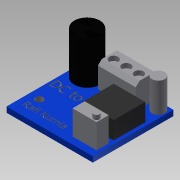
# Autodesk Inventor part: DC to DC
Saved by Autodesk Inventor 2015 SP1 (Build 190203100, 203)
## iProperties
Created: 2015-01-28
Part Number: DC to DC
Material: Generic
Document SubType Name: Modeling
Designer: Rafi Kurnia Putra
Density: 1 g/cm^3
Appearance: Default
Mass: 6.54094 g
Surface Area: 45.9552 cm^2
Volume: 6.54094 cm^3
Author: Rafi Kurnia Putra
Autodesk Inventor part; units mm, degrees
ref_plane "YZ Plane" through (0, 0, 0) normal (1, 0, 0) x (0, 1, 0)
ref_plane "XZ Plane" through (0, 0, 0) normal (0, 1, 0) x (-1, 0, 0)
ref_plane "XY Plane" through (0, 0, 0) normal (0, 0, 1) x (1, 0, 0)
sketch "Sketch1" plane through (0, 0, 0) normal (0, 1, 0) x (-1, 0, 0)
  line L0 (17.14, 16) -> (-17.14, 16)
  line L1 (-17.14, 16) -> (-17.14, -16)
  line L2 (-17.14, -16) -> (17.14, -16)
  line L3 (17.14, -16) -> (17.14, 16)
  line L4 (17.14, 16) -> (-17.14, -16) construction
  line L5 (-17.14, 16) -> (17.14, -16) construction
  circle A0 centre (13.09, 7.05) radius 1.5
  circle A1 centre (11.14, -10) radius 5.065
  circle A2 centre (2.4487, -11.859) radius 1.75
  circle A3 centre (-2.5513, -11.859) radius 1.75
  circle A4 centre (-7.5513, -11.859) radius 1.75
  circle A5 centre (-14.14, -13) radius 2.5
  line L6 (-3.3092, -6.109) -> (-15.8092, -6.109)
  line L7 (-15.8092, -6.109) -> (-15.8092, 6.391)
  line L8 (-15.8092, 6.391) -> (-3.3092, 6.391)
  line L9 (-3.3092, 6.391) -> (-3.3092, -6.109)
  line L10 (-3.3092, -6.109) -> (-15.8092, 6.391) construction
  line L11 (-15.8092, -6.109) -> (-3.3092, 6.391) construction
  line L12 (4.9487, -15.609) -> (-10.0513, -15.609)
  line L13 (-10.0513, -15.609) -> (-10.0513, -8.109)
  line L14 (-10.0513, -8.109) -> (4.9487, -8.109)
  line L15 (4.9487, -8.109) -> (4.9487, -15.609)
  line L16 (4.9487, -15.609) -> (-10.0513, -8.109) construction
  line L17 (-10.0513, -15.609) -> (4.9487, -8.109) construction
  line L18 (-6.279, 8.3837) -> (-15.809, 8.3837)
  line L19 (-15.809, 8.3837) -> (-15.809, 13.2037)
  line L20 (-15.809, 13.2037) -> (-6.279, 13.2037)
  line L21 (-6.279, 13.2037) -> (-6.279, 8.3837)
  line L22 (-6.279, 8.3837) -> (-15.809, 13.2037) construction
  line L23 (-15.809, 8.3837) -> (-6.279, 13.2037) construction
  circle A6 centre (-14.309, 11.7037) radius 1.155
  point P0 (0, 0)
  point P1 (-9.5592, 0.141)
  point P2 (-2.5513, -11.859)
  point P3 (-11.044, 10.7937)
  point P4 (-9.5592, 0.141)
  dimension "d0" = 34.28
  dimension "d1" = 32
  dimension "d2" = 3
  dimension "d3" = 4.05
  dimension "d4" = 8.95
  dimension "d5" = 10.13
  dimension "d6" = 6
  dimension "d7" = 6
  dimension "d8" = 3.5
  dimension "d9" = 3.5
  dimension "d10" = 3.5
  dimension "d11" = 5
  dimension "d12" = 5
  dimension "d13" = 5
  dimension "d14" = 3
  dimension "d15" = 3
  dimension "d16" = 12.5
  dimension "d17" = 12.5
  dimension "d18" = 15
  dimension "d19" = 7.5
  dimension "d20" = 2
  dimension "d21" = 9.53
  dimension "d22" = 4.82
  dimension "d23" = 1.3308
  dimension "d24" = 1.331
  dimension "d42" = 2.31
  dimension "d43" = 1.5
  dimension "d44" = 1.5
  constraints: 48 end point, 9 midpoint, 8 parallel, 7 centre point, 4 horizontal, 4 perpendicular, 1 other
  measures "d0" distance of L2.end L1.end
  measures "d1" distance of L1.end L0.end
  measures "d2" diameter of A0
  measures "d3" distance from line of A0.centre L3
  measures "d4" distance from line of L0 A0.centre
  measures "d5" diameter of A1
  measures "d6" distance from line of A1.centre L3
  measures "d7" distance from line of L2 A1.centre
  measures "d8" diameter of A2
  measures "d9" diameter of A3
  measures "d10" diameter of A4
  measures "d11" distance of A3.centre A2.centre
  measures "d12" distance of A4.centre A3.centre
  measures "d13" diameter of A5
  measures "d14" distance from line of A5.centre L2
  measures "d15" distance from line of L1 A5.centre
  measures "d16" distance of L7.end L8.end
  measures "d17" distance of L6.end L7.end
  measures "d18" distance of L13.end L14.end
  measures "d19" distance of L12.end L13.end
  measures "d20" distance between parallel lines of L6 L14
  measures "d21" distance of L19.end L20.end
  measures "d22" distance of L18.end L19.end
  measures "d23" distance between parallel lines of L1 L7
  measures "d24" distance between parallel lines of L1 L19
  measures "d42" diameter of A6
  measures "d43" distance from line of A6.centre L20
  measures "d44" distance from line of L19 A6.centre
extrude "Extrusion1" add sketch "Sketch1" along normal blind 2.15 contours L3 L2 L1 L0 | A1 | A2 | A3 | A4 | A5 | L6 L7 L8 L9 | L12 L13 L14 L15 | L18 L19 L20 L21 | A6
extrude "Extrusion2" add sketch "Sketch1" along normal blind 19.17 contours A1
extrude "Extrusion3" add sketch "Sketch1" along normal blind 11.77 contours L12 L13 L14 L15
chamfer "Chamfer1" distance 1.5 angle 45 1 edges at (2.5513, 11.77, -8.109)
extrude "Extrusion4" add sketch "Sketch1" along normal blind 10 contours A2 | A3 | A4
extrude "Extrusion5" add sketch "Sketch1" along normal blind 13.91 contours A5
extrude "Extrusion6" add sketch "Sketch1" along normal blind 9.14 contours L6 L7 L8 L9
extrude "Extrusion7" add sketch "Sketch1" along normal blind 11.85 contours L18 L19 L20 L21 | A6
extrude "Extrusion8" add sketch "Sketch1" along normal blind 13.61 contours A6
extrude "Extrusion9" add sketch "Sketch1" against normal blind 2.4 contours A2 | A3 | A4
sketch "Sketch2" plane through (0, 2.15, 0) normal (0, 1, 0) x (1, 0, 0)
  line L0 (-16.4252, 3.2471) -> (3.1141, 3.2471) construction
  line L1 (3.1141, 3.2471) -> (3.1141, -0.3891) construction
  line L2 (3.1141, -0.3891) -> (-16.4252, -0.3891) construction
  line L3 (-16.4252, -0.3891) -> (-16.4252, 3.2471) construction
  line L4 (-14.8497, -9.856) -> (21.0749, -9.856) construction
  line L5 (21.0749, -9.856) -> (21.0749, -13.6084) construction
  line L6 (21.0749, -13.6084) -> (-14.8497, -13.6084) construction
  line L7 (-14.8497, -13.6084) -> (-14.8497, -9.856) construction
  line L8 (-12.6267, -12.5257) -> (-13.0651, -12.5257)
  line L9 (-13.0651, -12.5257) -> (-13.8679, -11.515)
  line L10 (-13.8679, -11.515) -> (-14.2549, -11.515)
  line L11 (-14.2549, -11.515) -> (-14.2549, -12.5257)
  line L12 (-14.2549, -12.5257) -> (-14.5924, -12.5257)
  line L13 (-14.5924, -12.5257) -> (-14.5924, -9.9857)
  line L14 (-14.5924, -9.9857) -> (-13.9379, -9.9857)
  spline S0 degree 2 poles (-13.9379, -9.9857) (-13.7197, -9.9857) (-13.4253, -10.033) (-13.2916, -10.1195) knots 0 0 0 1 2 2 2
  spline S1 degree 2 poles (-13.2916, -10.1195) (-13.1578, -10.2059) (-13.0034, -10.4756) (-13.0034, -10.6752) knots 0 0 0 1 2 2 2
  spline S2 degree 2 poles (-13.0034, -10.6752) (-13.0034, -10.9531) (-13.2874, -11.3298) (-13.5303, -11.4204) knots 0 0 0 1 2 2 2
  line L15 (-13.5303, -11.4204) -> (-12.6267, -12.5257)
  spline S3 degree 2 poles (-13.3554, -10.702) (-13.3554, -10.5908) (-13.4336, -10.42) (-13.5159, -10.3644) knots 0 0 0 1 2 2 2
  spline S4 degree 2 poles (-13.5159, -10.3644) (-13.588, -10.3171) (-13.7794, -10.278) (-13.9193, -10.278) knots 0 0 0 1 2 2 2
  line L16 (-13.9193, -10.278) -> (-14.2549, -10.278)
  line L17 (-14.2549, -10.278) -> (-14.2549, -11.233)
  line L18 (-14.2549, -11.233) -> (-13.9585, -11.233)
  spline S5 degree 2 poles (-13.9585, -11.233) (-13.8123, -11.233) (-13.5797, -11.1816) (-13.4994, -11.1013) knots 0 0 0 1 2 2 2
  spline S6 degree 2 poles (-13.4994, -11.1013) (-13.4253, -11.0313) (-13.3554, -10.8337) (-13.3554, -10.702) knots 0 0 0 1 2 2 2
  spline S7 degree 2 poles (-11.3876, -12.324) (-11.4267, -12.3528) (-11.5584, -12.4557) (-11.6202, -12.4866) knots 0 0 0 1 2 2 2
  spline S8 degree 2 poles (-11.6202, -12.4866) (-11.7046, -12.5319) (-11.8631, -12.5792) (-12.0071, -12.5792) knots 0 0 0 1 2 2 2
  spline S9 degree 2 poles (-12.0071, -12.5792) (-12.1245, -12.5792) (-12.3365, -12.4907) (-12.4168, -12.4104) knots 0 0 0 1 2 2 2
  spline S10 degree 2 poles (-12.4168, -12.4104) (-12.4929, -12.3322) (-12.5855, -12.1017) (-12.5855, -11.974) knots 0 0 0 1 2 2 2
  spline S11 degree 2 poles (-12.5855, -11.974) (-12.5855, -11.7764) (-12.4188, -11.4965) (-12.2377, -11.4162) knots 0 0 0 1 2 2 2
  spline S12 degree 2 poles (-12.2377, -11.4162) (-12.0771, -11.3421) (-11.6408, -11.2866) (-11.3876, -11.2722) knots 0 0 0 1 2 2 2
  line L19 (-11.3876, -11.2722) -> (-11.3876, -11.2104)
  spline S13 degree 2 poles (-11.3876, -11.2104) (-11.3876, -11.0993) (-11.4555, -10.9613) (-11.5173, -10.9222) knots 0 0 0 1 2 2 2
  spline S14 degree 2 poles (-11.5173, -10.9222) (-11.579, -10.8831) (-11.756, -10.8584) (-11.8507, -10.8584) knots 0 0 0 1 2 2 2
  spline S15 degree 2 poles (-11.8507, -10.8584) (-11.9619, -10.8584) (-12.2624, -10.9243) (-12.4126, -10.9881) knots 0 0 0 1 2 2 2
  line L20 (-12.4126, -10.9881) -> (-12.4312, -10.9881)
  line L21 (-12.4312, -10.9881) -> (-12.4312, -10.6608)
  spline S16 degree 2 poles (-12.4312, -10.6608) (-12.3427, -10.6361) (-12.0113, -10.5744) (-11.8486, -10.5744) knots 0 0 0 1 2 2 2
  spline S17 degree 2 poles (-11.8486, -10.5744) (-11.651, -10.5744) (-11.3814, -10.6361) (-11.2744, -10.7164) knots 0 0 0 1 2 2 2
  spline S18 degree 2 poles (-11.2744, -10.7164) (-11.1694, -10.7946) (-11.0665, -11.0437) (-11.0665, -11.2228) knots 0 0 0 1 2 2 2
  line L22 (-11.0665, -11.2228) -> (-11.0665, -12.5257)
  line L23 (-11.0665, -12.5257) -> (-11.3876, -12.5257)
  line L24 (-11.3876, -12.5257) -> (-11.3876, -12.324)
  line L25 (-11.3876, -12.0564) -> (-11.3876, -11.5274)
  spline S19 degree 2 poles (-11.3876, -11.5274) (-11.5028, -11.5377) (-11.8507, -11.5727) (-11.9598, -11.6056) knots 0 0 0 1 2 2 2
  spline S20 degree 2 poles (-11.9598, -11.6056) (-12.0874, -11.6447) (-12.2541, -11.8073) (-12.2541, -11.9514) knots 0 0 0 1 2 2 2
  spline S21 degree 2 poles (-12.2541, -11.9514) (-12.2541, -12.1161) (-12.0689, -12.2828) (-11.8919, -12.2828) knots 0 0 0 1 2 2 2
  spline S22 degree 2 poles (-11.8919, -12.2828) (-11.7416, -12.2828) (-11.4946, -12.1531) (-11.3876, -12.0564) knots 0 0 0 1 2 2 2
  line L26 (-9.6133, -10.1812) -> (-9.6298, -10.1812)
  spline S23 degree 2 poles (-9.6298, -10.1812) (-9.673, -10.1648) (-9.8335, -10.1359) (-9.8973, -10.1359) knots 0 0 0 1 2 2 2
  spline S24 degree 2 poles (-9.8973, -10.1359) (-10.0991, -10.1359) (-10.272, -10.3171) (-10.272, -10.5558) knots 0 0 0 1 2 2 2
  line L27 (-10.272, -10.5558) -> (-10.272, -10.6197)
  line L28 (-10.272, -10.6197) -> (-9.7409, -10.6197)
  line L29 (-9.7409, -10.6197) -> (-9.7409, -10.8852)
  line L30 (-9.7409, -10.8852) -> (-10.2617, -10.8852)
  line L31 (-10.2617, -10.8852) -> (-10.2617, -12.5257)
  line L32 (-10.2617, -12.5257) -> (-10.5828, -12.5257)
  line L33 (-10.5828, -12.5257) -> (-10.5828, -10.8852)
  line L34 (-10.5828, -10.8852) -> (-10.7989, -10.8852)
  line L35 (-10.7989, -10.8852) -> (-10.7989, -10.6197)
  line L36 (-10.7989, -10.6197) -> (-10.5828, -10.6197)
  line L37 (-10.5828, -10.6197) -> (-10.5828, -10.5558)
  spline S25 degree 2 poles (-10.5828, -10.5558) (-10.5828, -10.2142) (-10.2514, -9.856) (-9.9426, -9.856) knots 0 0 0 1 2 2 2
  spline S26 degree 2 poles (-9.9426, -9.856) (-9.8541, -9.856) (-9.6833, -9.8745) (-9.6133, -9.8869) knots 0 0 0 1 2 2 2
  line L38 (-9.6133, -9.8869) -> (-9.6133, -10.1812)
  line L39 (-9.1769, -12.5257) -> (-9.498, -12.5257)
  line L40 (-9.498, -12.5257) -> (-9.498, -10.6197)
  line L41 (-9.498, -10.6197) -> (-9.1769, -10.6197)
  line L42 (-9.1769, -10.6197) -> (-9.1769, -12.5257)
  line L43 (-9.1543, -10.3027) -> (-9.5186, -10.3027)
  line L44 (-9.5186, -10.3027) -> (-9.5186, -9.9692)
  line L45 (-9.5186, -9.9692) -> (-9.1543, -9.9692)
  line L46 (-9.1543, -9.9692) -> (-9.1543, -10.3027)
  line L47 (-5.7374, -12.5257) -> (-6.1758, -12.5257)
  line L48 (-6.1758, -12.5257) -> (-7.1042, -11.3442)
  line L49 (-7.1042, -11.3442) -> (-7.2524, -11.5109)
  line L50 (-7.2524, -11.5109) -> (-7.2524, -12.5257)
  line L51 (-7.2524, -12.5257) -> (-7.5899, -12.5257)
  line L52 (-7.5899, -12.5257) -> (-7.5899, -9.9857)
  line L53 (-7.5899, -9.9857) -> (-7.2524, -9.9857)
  line L54 (-7.2524, -9.9857) -> (-7.2524, -11.1528)
  line L55 (-7.2524, -11.1528) -> (-6.2108, -9.9857)
  line L56 (-6.2108, -9.9857) -> (-5.7992, -9.9857)
  line L57 (-5.7992, -9.9857) -> (-6.851, -11.1198)
  line L58 (-6.851, -11.1198) -> (-5.7374, -12.5257)
  line L59 (-4.0784, -12.5257) -> (-4.3995, -12.5257)
  line L60 (-4.3995, -12.5257) -> (-4.3995, -12.3157)
  spline S27 degree 2 poles (-4.3995, -12.3157) (-4.5477, -12.4454) (-4.8132, -12.5792) (-4.9779, -12.5792) knots 0 0 0 1 2 2 2
  spline S28 degree 2 poles (-4.9779, -12.5792) (-5.1014, -12.5792) (-5.3216, -12.4969) (-5.4019, -12.4084) knots 0 0 0 1 2 2 2
  spline S29 degree 2 poles (-5.4019, -12.4084) (-5.4842, -12.3199) (-5.5748, -12.0502) (-5.5748, -11.8567) knots 0 0 0 1 2 2 2
  line L61 (-5.5748, -11.8567) -> (-5.5748, -10.6197)
  line L62 (-5.5748, -10.6197) -> (-5.2537, -10.6197)
  line L63 (-5.2537, -10.6197) -> (-5.2537, -11.7065)
  spline S30 degree 2 poles (-5.2537, -11.7065) (-5.2537, -11.8588) (-5.2311, -12.0584) (-5.192, -12.1325) knots 0 0 0 1 2 2 2
  spline S31 degree 2 poles (-5.192, -12.1325) (-5.1528, -12.2066) (-5.0191, -12.2746) (-4.8935, -12.2746) knots 0 0 0 1 2 2 2
  spline S32 degree 2 poles (-4.8935, -12.2746) (-4.7762, -12.2746) (-4.5106, -12.1408) (-4.3995, -12.044) knots 0 0 0 1 2 2 2
  line L64 (-4.3995, -12.044) -> (-4.3995, -10.6197)
  line L65 (-4.3995, -10.6197) -> (-4.0784, -10.6197)
  line L66 (-4.0784, -10.6197) -> (-4.0784, -12.5257)
  line L67 (-2.6026, -10.9634) -> (-2.619, -10.9634)
  spline S33 degree 2 poles (-2.619, -10.9634) (-2.6561, -10.9531) (-2.7363, -10.949) (-2.7919, -10.949) knots 0 0 0 1 2 2 2
  spline S34 degree 2 poles (-2.7919, -10.949) (-2.9216, -10.949) (-3.1768, -11.0622) (-3.2921, -11.1734) knots 0 0 0 1 2 2 2
  line L68 (-3.2921, -11.1734) -> (-3.2921, -12.5257)
  line L69 (-3.2921, -12.5257) -> (-3.6132, -12.5257)
  line L70 (-3.6132, -12.5257) -> (-3.6132, -10.6197)
  line L71 (-3.6132, -10.6197) -> (-3.2921, -10.6197)
  line L72 (-3.2921, -10.6197) -> (-3.2921, -10.9037)
  spline S35 degree 2 poles (-3.2921, -10.9037) (-3.1171, -10.7473) (-2.8557, -10.6197) (-2.7322, -10.6197) knots 0 0 0 1 2 2 2
  spline S36 degree 2 poles (-2.7322, -10.6197) (-2.6828, -10.6197) (-2.6334, -10.6238) (-2.6026, -10.6299) knots 0 0 0 1 2 2 2
  line L73 (-2.6026, -10.6299) -> (-2.6026, -10.9634)
  line L74 (-0.8571, -12.5257) -> (-1.1782, -12.5257)
  line L75 (-1.1782, -12.5257) -> (-1.1782, -11.4389)
  spline S37 degree 2 poles (-1.1782, -11.4389) (-1.1782, -11.3071) (-1.2029, -11.0807) (-1.2399, -11.0128) knots 0 0 0 1 2 2 2
  spline S38 degree 2 poles (-1.2399, -11.0128) (-1.279, -10.9408) (-1.419, -10.8708) (-1.5384, -10.8708) knots 0 0 0 1 2 2 2
  spline S39 degree 2 poles (-1.5384, -10.8708) (-1.6578, -10.8708) (-1.911, -10.9984) (-2.0324, -11.1013) knots 0 0 0 1 2 2 2
  line L76 (-2.0324, -11.1013) -> (-2.0324, -12.5257)
  line L77 (-2.0324, -12.5257) -> (-2.3535, -12.5257)
  line L78 (-2.3535, -12.5257) -> (-2.3535, -10.6197)
  line L79 (-2.3535, -10.6197) -> (-2.0324, -10.6197)
  line L80 (-2.0324, -10.6197) -> (-2.0324, -10.8317)
  spline S40 degree 2 poles (-2.0324, -10.8317) (-1.8883, -10.702) (-1.6104, -10.5661) (-1.454, -10.5661) knots 0 0 0 1 2 2 2
  spline S41 degree 2 poles (-1.454, -10.5661) (-1.1741, -10.5661) (-0.8571, -10.9366) (-0.8571, -11.2886) knots 0 0 0 1 2 2 2
  line L81 (-0.8571, -11.2886) -> (-0.8571, -12.5257)
  line L82 (-0.079, -12.5257) -> (-0.4001, -12.5257)
  line L83 (-0.4001, -12.5257) -> (-0.4001, -10.6197)
  line L84 (-0.4001, -10.6197) -> (-0.079, -10.6197)
  line L85 (-0.079, -10.6197) -> (-0.079, -12.5257)
  line L86 (-0.0564, -10.3027) -> (-0.4207, -10.3027)
  line L87 (-0.4207, -10.3027) -> (-0.4207, -9.9692)
  line L88 (-0.4207, -9.9692) -> (-0.0564, -9.9692)
  line L89 (-0.0564, -9.9692) -> (-0.0564, -10.3027)
  spline S42 degree 2 poles (1.4544, -12.324) (1.4153, -12.3528) (1.2836, -12.4557) (1.2219, -12.4866) knots 0 0 0 1 2 2 2
  spline S43 degree 2 poles (1.2219, -12.4866) (1.1375, -12.5319) (0.979, -12.5792) (0.8349, -12.5792) knots 0 0 0 1 2 2 2
  spline S44 degree 2 poles (0.8349, -12.5792) (0.7176, -12.5792) (0.5055, -12.4907) (0.4253, -12.4104) knots 0 0 0 1 2 2 2
  spline S45 degree 2 poles (0.4253, -12.4104) (0.3491, -12.3322) (0.2565, -12.1017) (0.2565, -11.974) knots 0 0 0 1 2 2 2
  spline S46 degree 2 poles (0.2565, -11.974) (0.2565, -11.7764) (0.4232, -11.4965) (0.6043, -11.4162) knots 0 0 0 1 2 2 2
  spline S47 degree 2 poles (0.6043, -11.4162) (0.7649, -11.3421) (1.2013, -11.2866) (1.4544, -11.2722) knots 0 0 0 1 2 2 2
  line L90 (1.4544, -11.2722) -> (1.4544, -11.2104)
  spline S48 degree 2 poles (1.4544, -11.2104) (1.4544, -11.0993) (1.3865, -10.9613) (1.3248, -10.9222) knots 0 0 0 1 2 2 2
  spline S49 degree 2 poles (1.3248, -10.9222) (1.263, -10.8831) (1.086, -10.8584) (0.9913, -10.8584) knots 0 0 0 1 2 2 2
  spline S50 degree 2 poles (0.9913, -10.8584) (0.8802, -10.8584) (0.5796, -10.9243) (0.4294, -10.9881) knots 0 0 0 1 2 2 2
  line L91 (0.4294, -10.9881) -> (0.4109, -10.9881)
  line L92 (0.4109, -10.9881) -> (0.4109, -10.6608)
  spline S51 degree 2 poles (0.4109, -10.6608) (0.4994, -10.6361) (0.8308, -10.5744) (0.9934, -10.5744) knots 0 0 0 1 2 2 2
  spline S52 degree 2 poles (0.9934, -10.5744) (1.191, -10.5744) (1.4606, -10.6361) (1.5677, -10.7164) knots 0 0 0 1 2 2 2
  spline S53 degree 2 poles (1.5677, -10.7164) (1.6726, -10.7946) (1.7755, -11.0437) (1.7755, -11.2228) knots 0 0 0 1 2 2 2
  line L93 (1.7755, -11.2228) -> (1.7755, -12.5257)
  line L94 (1.7755, -12.5257) -> (1.4544, -12.5257)
  line L95 (1.4544, -12.5257) -> (1.4544, -12.324)
  line L96 (1.4544, -12.0564) -> (1.4544, -11.5274)
  spline S54 degree 2 poles (1.4544, -11.5274) (1.3392, -11.5377) (0.9913, -11.5727) (0.8822, -11.6056) knots 0 0 0 1 2 2 2
  spline S55 degree 2 poles (0.8822, -11.6056) (0.7546, -11.6447) (0.5879, -11.8073) (0.5879, -11.9514) knots 0 0 0 1 2 2 2
  spline S56 degree 2 poles (0.5879, -11.9514) (0.5879, -12.1161) (0.7731, -12.2828) (0.9502, -12.2828) knots 0 0 0 1 2 2 2
  spline S57 degree 2 poles (0.9502, -12.2828) (1.1004, -12.2828) (1.3474, -12.1531) (1.4544, -12.0564) knots 0 0 0 1 2 2 2
  spline S58 degree 2 poles (-13.311, 1.4318) (-13.311, 0.9525) (-13.6996, 0.181) (-14.0257, -0.0345) knots 0 0 0 1 2 2 2
  spline S59 degree 2 poles (-14.0257, -0.0345) (-14.2923, -0.2019) (-14.8397, -0.3153) (-15.2652, -0.3153) knots 0 0 0 1 2 2 2
  line L97 (-15.2652, -0.3153) -> (-16.0707, -0.3153)
  line L98 (-16.0707, -0.3153) -> (-16.0707, 3.1847)
  line L99 (-16.0707, 3.1847) -> (-15.2737, 3.1847)
  spline S60 degree 2 poles (-15.2737, 3.1847) (-14.7802, 3.1847) (-14.2186, 3.0372) (-14.0201, 2.9067) knots 0 0 0 1 2 2 2
  spline S61 degree 2 poles (-14.0201, 2.9067) (-13.6825, 2.6827) (-13.311, 1.9424) (-13.311, 1.4318) knots 0 0 0 1 2 2 2
  spline S62 degree 2 poles (-13.796, 1.4375) (-13.796, 1.8403) (-14.0626, 2.4104) (-14.3264, 2.572) knots 0 0 0 1 2 2 2
  spline S63 degree 2 poles (-14.3264, 2.572) (-14.5136, 2.6827) (-14.9362, 2.7819) (-15.251, 2.7819) knots 0 0 0 1 2 2 2
  line L100 (-15.251, 2.7819) -> (-15.6056, 2.7819)
  line L101 (-15.6056, 2.7819) -> (-15.6056, 0.0874)
  line L102 (-15.6056, 0.0874) -> (-15.251, 0.0874)
  spline S64 degree 2 poles (-15.251, 0.0874) (-14.9419, 0.0874) (-14.4739, 0.1867) (-14.2838, 0.32) knots 0 0 0 1 2 2 2
  spline S65 degree 2 poles (-14.2838, 0.32) (-14.0399, 0.4845) (-13.796, 1.0291) (-13.796, 1.4375) knots 0 0 0 1 2 2 2
  spline S66 degree 2 poles (-11.439, -0.3777) (-11.7794, -0.3777) (-12.3551, -0.148) (-12.565, 0.0818) knots 0 0 0 1 2 2 2
  spline S67 degree 2 poles (-12.565, 0.0818) (-12.7749, 0.3087) (-13.0047, 0.9894) (-13.0047, 1.4318) knots 0 0 0 1 2 2 2
  spline S68 degree 2 poles (-13.0047, 1.4318) (-13.0047, 1.8715) (-12.7806, 2.5238) (-12.5679, 2.7649) knots 0 0 0 1 2 2 2
  spline S69 degree 2 poles (-12.5679, 2.7649) (-12.358, 3.0003) (-11.785, 3.2471) (-11.4305, 3.2471) knots 0 0 0 1 2 2 2
  spline S70 degree 2 poles (-11.4305, 3.2471) (-11.2547, 3.2471) (-10.9455, 3.196) (-10.815, 3.1563) knots 0 0 0 1 2 2 2
  spline S71 degree 2 poles (-10.815, 3.1563) (-10.7016, 3.1194) (-10.4662, 3.0145) (-10.3499, 2.9521) knots 0 0 0 1 2 2 2
  line L103 (-10.3499, 2.9521) -> (-10.3499, 2.3905)
  line L104 (-10.3499, 2.3905) -> (-10.3867, 2.3905)
  spline S72 degree 2 poles (-10.3867, 2.3905) (-10.4491, 2.4472) (-10.642, 2.6061) (-10.781, 2.6827) knots 0 0 0 1 2 2 2
  spline S73 degree 2 poles (-10.781, 2.6827) (-10.9143, 2.7564) (-11.2291, 2.85) (-11.4333, 2.85) knots 0 0 0 1 2 2 2
  spline S74 degree 2 poles (-11.4333, 2.85) (-11.6574, 2.85) (-12.0573, 2.6656) (-12.2077, 2.4898) knots 0 0 0 1 2 2 2
  spline S75 degree 2 poles (-12.2077, 2.4898) (-12.3551, 2.3111) (-12.5197, 1.7694) (-12.5197, 1.4318) knots 0 0 0 1 2 2 2
  spline S76 degree 2 poles (-12.5197, 1.4318) (-12.5197, 1.0716) (-12.3466, 0.5526) (-12.1963, 0.3739) knots 0 0 0 1 2 2 2
  spline S77 degree 2 poles (-12.1963, 0.3739) (-12.0488, 0.2009) (-11.6546, 0.025) (-11.4333, 0.025) knots 0 0 0 1 2 2 2
  spline S78 degree 2 poles (-11.4333, 0.025) (-11.232, 0.025) (-10.8888, 0.1243) (-10.7555, 0.1981) knots 0 0 0 1 2 2 2
  spline S79 degree 2 poles (-10.7555, 0.1981) (-10.6278, 0.2718) (-10.4378, 0.425) (-10.3839, 0.4789) knots 0 0 0 1 2 2 2
  line L105 (-10.3839, 0.4789) -> (-10.3499, 0.4789)
  line L106 (-10.3499, 0.4789) -> (-10.3499, -0.0771)
  spline S80 degree 2 poles (-10.3499, -0.0771) (-10.4662, -0.131) (-10.6704, -0.2302) (-10.815, -0.2756) knots 0 0 0 1 2 2 2
  spline S81 degree 2 poles (-10.815, -0.2756) (-10.9682, -0.3267) (-11.2291, -0.3777) (-11.439, -0.3777) knots 0 0 0 1 2 2 2
  spline S82 degree 2 poles (-7.6526, -0.3664) (-8.0128, -0.3664) (-8.4184, 0.0449) (-8.4184, 0.4902) knots 0 0 0 1 2 2 2
  line L107 (-8.4184, 0.4902) -> (-8.4184, 1.9452)
  line L108 (-8.4184, 1.9452) -> (-8.7162, 1.9452)
  line L109 (-8.7162, 1.9452) -> (-8.7162, 2.3111)
  line L110 (-8.7162, 2.3111) -> (-8.4184, 2.3111)
  line L111 (-8.4184, 2.3111) -> (-8.4184, 3.0656)
  line L112 (-8.4184, 3.0656) -> (-7.9759, 3.0656)
  line L113 (-7.9759, 3.0656) -> (-7.9759, 2.3111)
  line L114 (-7.9759, 2.3111) -> (-7.1619, 2.3111)
  line L115 (-7.1619, 2.3111) -> (-7.1619, 1.9452)
  line L116 (-7.1619, 1.9452) -> (-7.9759, 1.9452)
  line L117 (-7.9759, 1.9452) -> (-7.9759, 0.6944)
  spline S83 degree 2 poles (-7.9759, 0.6944) (-7.9759, 0.4959) (-7.9617, 0.2775) (-7.9135, 0.1839) knots 0 0 0 1 2 2 2
  spline S84 degree 2 poles (-7.9135, 0.1839) (-7.8738, 0.1016) (-7.6951, 0.0194) (-7.5419, 0.0194) knots 0 0 0 1 2 2 2
  spline S85 degree 2 poles (-7.5419, 0.0194) (-7.4342, 0.0194) (-7.2328, 0.0846) (-7.1874, 0.1045) knots 0 0 0 1 2 2 2
  line L118 (-7.1874, 0.1045) -> (-7.1619, 0.1045)
  line L119 (-7.1619, 0.1045) -> (-7.1619, -0.2926)
  spline S86 degree 2 poles (-7.1619, -0.2926) (-7.2867, -0.3267) (-7.5419, -0.3664) (-7.6526, -0.3664) knots 0 0 0 1 2 2 2
  spline S87 degree 2 poles (-4.6773, 0.9979) (-4.6773, 0.3342) (-5.3154, -0.3891) (-5.8487, -0.3891) knots 0 0 0 1 2 2 2
  spline S88 degree 2 poles (-5.8487, -0.3891) (-6.3961, -0.3891) (-7.0229, 0.3569) (-7.0229, 0.9979) knots 0 0 0 1 2 2 2
  spline S89 degree 2 poles (-7.0229, 0.9979) (-7.0229, 1.6559) (-6.3762, 2.3848) (-5.8487, 2.3848) knots 0 0 0 1 2 2 2
  spline S90 degree 2 poles (-5.8487, 2.3848) (-5.3154, 2.3848) (-4.6773, 1.6588) (-4.6773, 0.9979) knots 0 0 0 1 2 2 2
  spline S91 degree 2 poles (-5.1339, 0.9979) (-5.1339, 1.5084) (-5.5055, 2.0048) (-5.8487, 2.0048) knots 0 0 0 1 2 2 2
  spline S92 degree 2 poles (-5.8487, 2.0048) (-6.1919, 2.0048) (-6.5662, 1.5084) (-6.5662, 0.9979) knots 0 0 0 1 2 2 2
  spline S93 degree 2 poles (-6.5662, 0.9979) (-6.5662, 0.5015) (-6.1919, -0.009) (-5.8487, -0.009) knots 0 0 0 1 2 2 2
  spline S94 degree 2 poles (-5.8487, -0.009) (-5.5083, -0.009) (-5.1339, 0.493) (-5.1339, 0.9979) knots 0 0 0 1 2 2 2
  spline S95 degree 2 poles (0.0735, 1.4318) (0.0735, 0.9525) (-0.315, 0.181) (-0.6412, -0.0345) knots 0 0 0 1 2 2 2
  spline S96 degree 2 poles (-0.6412, -0.0345) (-0.9078, -0.2019) (-1.4552, -0.3153) (-1.8807, -0.3153) knots 0 0 0 1 2 2 2
  line L120 (-1.8807, -0.3153) -> (-2.6862, -0.3153)
  line L121 (-2.6862, -0.3153) -> (-2.6862, 3.1847)
  line L122 (-2.6862, 3.1847) -> (-1.8892, 3.1847)
  spline S97 degree 2 poles (-1.8892, 3.1847) (-1.3957, 3.1847) (-0.8341, 3.0372) (-0.6355, 2.9067) knots 0 0 0 1 2 2 2
  spline S98 degree 2 poles (-0.6355, 2.9067) (-0.298, 2.6827) (0.0735, 1.9424) (0.0735, 1.4318) knots 0 0 0 1 2 2 2
  spline S99 degree 2 poles (-0.4115, 1.4375) (-0.4115, 1.8403) (-0.6781, 2.4104) (-0.9419, 2.572) knots 0 0 0 1 2 2 2
  spline S100 degree 2 poles (-0.9419, 2.572) (-1.1291, 2.6827) (-1.5517, 2.7819) (-1.8665, 2.7819) knots 0 0 0 1 2 2 2
  line L123 (-1.8665, 2.7819) -> (-2.221, 2.7819)
  line L124 (-2.221, 2.7819) -> (-2.221, 0.0874)
  line L125 (-2.221, 0.0874) -> (-1.8665, 0.0874)
  spline S101 degree 2 poles (-1.8665, 0.0874) (-1.5573, 0.0874) (-1.0893, 0.1867) (-0.8993, 0.32) knots 0 0 0 1 2 2 2
  spline S102 degree 2 poles (-0.8993, 0.32) (-0.6554, 0.4845) (-0.4115, 1.0291) (-0.4115, 1.4375) knots 0 0 0 1 2 2 2
  spline S103 degree 2 poles (1.9455, -0.3777) (1.6051, -0.3777) (1.0294, -0.148) (0.8195, 0.0818) knots 0 0 0 1 2 2 2
  spline S104 degree 2 poles (0.8195, 0.0818) (0.6096, 0.3087) (0.3799, 0.9894) (0.3799, 1.4318) knots 0 0 0 1 2 2 2
  spline S105 degree 2 poles (0.3799, 1.4318) (0.3799, 1.8715) (0.6039, 2.5238) (0.8167, 2.7649) knots 0 0 0 1 2 2 2
  spline S106 degree 2 poles (0.8167, 2.7649) (1.0265, 3.0003) (1.5995, 3.2471) (1.954, 3.2471) knots 0 0 0 1 2 2 2
  spline S107 degree 2 poles (1.954, 3.2471) (2.1299, 3.2471) (2.439, 3.196) (2.5695, 3.1563) knots 0 0 0 1 2 2 2
  spline S108 degree 2 poles (2.5695, 3.1563) (2.6829, 3.1194) (2.9184, 3.0145) (3.0346, 2.9521) knots 0 0 0 1 2 2 2
  line L126 (3.0346, 2.9521) -> (3.0346, 2.3905)
  line L127 (3.0346, 2.3905) -> (2.9978, 2.3905)
  spline S109 degree 2 poles (2.9978, 2.3905) (2.9354, 2.4472) (2.7425, 2.6061) (2.6035, 2.6827) knots 0 0 0 1 2 2 2
  spline S110 degree 2 poles (2.6035, 2.6827) (2.4702, 2.7564) (2.1554, 2.85) (1.9512, 2.85) knots 0 0 0 1 2 2 2
  spline S111 degree 2 poles (1.9512, 2.85) (1.7271, 2.85) (1.3272, 2.6656) (1.1769, 2.4898) knots 0 0 0 1 2 2 2
  spline S112 degree 2 poles (1.1769, 2.4898) (1.0294, 2.3111) (0.8649, 1.7694) (0.8649, 1.4318) knots 0 0 0 1 2 2 2
  spline S113 degree 2 poles (0.8649, 1.4318) (0.8649, 1.0716) (1.0379, 0.5526) (1.1882, 0.3739) knots 0 0 0 1 2 2 2
  spline S114 degree 2 poles (1.1882, 0.3739) (1.3357, 0.2009) (1.7299, 0.025) (1.9512, 0.025) knots 0 0 0 1 2 2 2
  spline S115 degree 2 poles (1.9512, 0.025) (2.1526, 0.025) (2.4957, 0.1243) (2.6291, 0.1981) knots 0 0 0 1 2 2 2
  spline S116 degree 2 poles (2.6291, 0.1981) (2.7567, 0.2718) (2.9467, 0.425) (3.0006, 0.4789) knots 0 0 0 1 2 2 2
  line L128 (3.0006, 0.4789) -> (3.0346, 0.4789)
  line L129 (3.0346, 0.4789) -> (3.0346, -0.0771)
  spline S117 degree 2 poles (3.0346, -0.0771) (2.9184, -0.131) (2.7141, -0.2302) (2.5695, -0.2756) knots 0 0 0 1 2 2 2
  spline S118 degree 2 poles (2.5695, -0.2756) (2.4163, -0.3267) (2.1554, -0.3777) (1.9455, -0.3777) knots 0 0 0 1 2 2 2
  point P0 (0, 0)
  constraints: 4 other
extrude "Extrusion10" cut sketch "Sketch2" against normal blind 1
body "Solid1"
